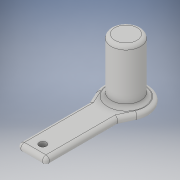
# Autodesk Inventor part: ConexionDireccionBottom
Saved by Autodesk Inventor 2019 (Build 230136000, 136)
## iProperties
Created: 2019-12-22
Part Number: ConexionDireccionBottom
Material: Generic
Document SubType Name: Modeling
Designer: Sergio
Density: 1 g/cm^3
Appearance: Default
Author: Sergio
Autodesk Inventor part; units mm, degrees
ref_plane "YZ Plane" through (0, 0, 0) normal (1, 0, 0) x (0, 1, 0)
ref_plane "XZ Plane" through (0, 0, 0) normal (0, 1, 0) x (-1, 0, 0)
ref_plane "XY Plane" through (0, 0, 0) normal (0, 0, 1) x (1, 0, 0)
sketch "Sketch1" plane through (0, 0, 0) normal (1, 0, 0) x (0, 1, 0)
  line L0 (14, 0) -> (14, -4)
  line L1 (14, -4) -> (0, -4)
  line L2 (0, -4) -> (0, -10.6835)
  line L3 (0, -10.6835) -> (4, -10.6835)
  line L4 (4, -10.6835) -> (4, -8.15)
  line L5 (4, -8.15) -> (34, -8.15)
  line L6 (34, -8.15) -> (34, 0)
  line L7 (34, 0) -> (14, 0)
  line L8 (49.6921, 0) -> (-25.5343, 0) construction
  point P0 (0, 0)
  dimension "d0" = 14
  dimension "d1" = 0
  dimension "d2" = 8.15
  dimension "d3" = 4
  dimension "d4" = 30
  dimension "d5" = 4
  constraints: 18 end point, 7 perpendicular, 1 horizontal, 1 vertical
  measures "d0" distance from line of point (0, 0) L0
  measures "d1" distance from line of point (0, 0) L2
  measures "d2" distance from line of point (0, 0) L5
  measures "d3" distance from line of point (0, 0) L1
  measures "d4" distance of L4.end L5.end
  measures "d5" distance of L2.end L3.end
revolve "Revolution1" add sketch "Sketch1" angle 360 about axis through (0, 49.6921, 0) along (0, -1, 0)
sketch "Sketch2" plane through (0, 0, 0) normal (0, 1, 0) x (-1, 0, 0)
  circle A0 centre (0, 0) radius 10
  arc A1 (-11.3543, 5.2278) -> (11.3543, 5.2278) centre (0, 0) ccw
  line L0 (8, 52.5131) -> (-8, 52.5131)
  line L1 (-8, 52.5131) -> (-8, 12.5131)
  line L2 (8, 12.5131) -> (8, 52.5131)
  circle A2 centre (0, 46.2702) radius 2
  line L3 (8, 12.5131) -> (11.3543, 5.2278)
  line L4 (-8, 12.5131) -> (-11.3543, 5.2278)
  dimension "d7" = 20
  dimension "d9" = 25
  dimension "d10" = 16
  dimension "d11" = 40
  dimension "d12" = 8
  dimension "d19" = 4
  constraints: 10 end point, 3 centre point, 2 point on circle, 2 tangent, 1 coincident, 1 horizontal, 1 parallel, 1 perpendicular
  measures "d7" diameter of A0
  measures "d9" diameter of A1
  measures "d10" distance of L2.start L1.end
  measures "d11" distance of L1.end L0.end
  measures "d12" distance from line of point (0, 0) L2
  measures "d19" diameter of A2
extrude "Extrusion1" add sketch "Sketch2" along normal blind 4
fillet "Fillet1" radius 2 13 edges at (0, 4, 52.5131) (8, 4, 32.5131) (-8, 4, 32.5131) (8, 0, 32.5131) (0, 0, 52.5131) (-9.6772, 0, 8.8704) (9.6772, 0, 8.8704) (0, 0, -12.5) (-9.6772, 4, 8.8704) (9.6772, 4, 8.8704) (0, 4, -12.5) (-8, 0, 32.5131) (0, 4, 8.15)
fillet "Fillet2" radius 2 1 edges at (0, 34, 8.15)
fillet "Fillet3" radius 2 6 edges at (-7.4142, 3.4142, 51.9273) (-8, 2, 52.5131) (-7.4142, 0.5858, 51.9273) (7.4142, 3.4142, 51.9273) (8, 2, 52.5131) (7.4142, 0.5858, 51.9273)
body "Solid1"
